minecraftdiamondsword .3 mm with all correct_v4 (Autodesk Fusion 360 design; units mm, degrees)
Autodesk Fusion 360 part; units mm, degrees
sketch "center" plane through (0, 0, 0) normal (0, 0, 1) x (1, 0, 0)
  line L0 (0, 22.6274) -> (2.8284, 19.799)
  line L1 (2.8284, 19.799) -> (5.6569, 22.6274)
  line L2 (5.6569, 22.6274) -> (2.8284, 25.4558)
  line L3 (2.8284, 25.4558) -> (0, 22.6274)
  line L4 (5.6569, 22.6274) -> (8.4853, 19.799)
  line L5 (8.4853, 19.799) -> (11.3137, 22.6274)
  line L6 (11.3137, 22.6274) -> (8.4853, 25.4558)
  line L7 (8.4853, 25.4558) -> (5.6569, 22.6274)
  line L8 (11.3137, 22.6274) -> (14.1421, 19.799)
  line L9 (14.1421, 19.799) -> (16.9706, 22.6274)
  line L10 (16.9706, 22.6274) -> (14.1421, 25.4558)
  line L11 (14.1421, 25.4558) -> (11.3137, 22.6274)
  line L12 (16.9706, 22.6274) -> (19.799, 19.799)
  line L13 (19.799, 19.799) -> (22.6274, 22.6274)
  line L14 (22.6274, 22.6274) -> (19.799, 25.4558)
  line L15 (19.799, 25.4558) -> (16.9706, 22.6274)
  line L16 (22.6274, 22.6274) -> (25.4558, 19.799)
  line L17 (25.4558, 19.799) -> (28.2843, 22.6274)
  line L18 (28.2843, 22.6274) -> (25.4558, 25.4558)
  line L19 (25.4558, 25.4558) -> (22.6274, 22.6274)
  line L20 (28.2843, 22.6274) -> (31.1127, 19.799)
  line L21 (31.1127, 19.799) -> (33.9411, 22.6274)
  line L22 (33.9411, 22.6274) -> (31.1127, 25.4558)
  line L23 (31.1127, 25.4558) -> (28.2843, 22.6274)
  line L24 (33.9411, 22.6274) -> (36.7696, 19.799)
  line L25 (36.7696, 19.799) -> (39.598, 22.6274)
  line L26 (39.598, 22.6274) -> (36.7696, 25.4558)
  line L27 (36.7696, 25.4558) -> (33.9411, 22.6274)
  line L28 (39.598, 22.6274) -> (42.4264, 19.799)
  line L29 (42.4264, 19.799) -> (45.2548, 22.6274)
  line L30 (45.2548, 22.6274) -> (42.4264, 25.4558)
  line L31 (42.4264, 25.4558) -> (39.598, 22.6274)
  line L32 (45.2548, 22.6274) -> (48.0833, 19.799)
  line L33 (48.0833, 19.799) -> (50.9117, 22.6274)
  line L34 (50.9117, 22.6274) -> (48.0833, 25.4558)
  line L35 (48.0833, 25.4558) -> (45.2548, 22.6274)
  line L36 (50.9117, 22.6274) -> (53.7401, 19.799)
  line L37 (53.7401, 19.799) -> (56.5685, 22.6274)
  line L38 (56.5685, 22.6274) -> (53.7401, 25.4558)
  line L39 (53.7401, 25.4558) -> (50.9117, 22.6274)
  line L40 (62.2254, 22.6274) -> (59.397, 25.4558)
  line L41 (70.7107, 25.4558) -> (67.8823, 22.6274)
  line L42 (90.5097, 22.6274) -> (87.6812, 25.4558)
  line L43 (62.2254, 22.6274) -> (65.0538, 19.799)
  line L44 (79.196, 22.6274) -> (76.3675, 25.4558)
  line L45 (84.8528, 22.6274) -> (87.6812, 19.799)
  line L46 (82.0244, 25.4558) -> (79.196, 22.6274)
  line L47 (76.3675, 25.4558) -> (73.5391, 22.6274)
  line L48 (87.6812, 25.4558) -> (84.8528, 22.6274)
  line L49 (73.5391, 22.6274) -> (76.3675, 19.799)
  line L50 (79.196, 22.6274) -> (82.0244, 19.799)
  line L51 (67.8823, 22.6274) -> (65.0538, 25.4558)
  line L52 (67.8823, 22.6274) -> (70.7107, 19.799)
  line L53 (76.3675, 19.799) -> (79.196, 22.6274)
  line L54 (59.397, 19.799) -> (62.2254, 22.6274)
  line L55 (56.5685, 22.6274) -> (59.397, 19.799)
  line L56 (59.397, 25.4558) -> (56.5685, 22.6274)
  line L57 (84.8528, 22.6274) -> (82.0244, 25.4558)
  line L58 (73.5391, 22.6274) -> (70.7107, 25.4558)
  line L59 (65.0538, 19.799) -> (67.8823, 22.6274)
  line L60 (87.6812, 19.799) -> (90.5097, 22.6274)
  line L61 (65.0538, 25.4558) -> (62.2254, 22.6274)
  line L62 (70.7107, 19.799) -> (73.5391, 22.6274)
  line L63 (82.0244, 19.799) -> (84.8528, 22.6274)
  dimension "d28" = 4
  dimension "d29" = 4
  dimension "d30" = 4
  dimension "d31" = 4
  dimension "d32" = 4
  dimension "d33" = 4
  dimension "d34" = 4
  dimension "d35" = 4
  dimension "d36" = 4
  dimension "d37" = 4
  dimension "d38" = 4
  dimension "d39" = 4
  dimension "d40" = 4
  dimension "d41" = 4
  dimension "d42" = 4
  dimension "d43" = 4
  dimension "d44" = 4
  dimension "d45" = 4
  dimension "d46" = 4
  dimension "d47" = 4
  dimension "d48" = 4
  dimension "d49" = 4
  dimension "d50" = 4
  dimension "d51" = 4
  dimension "d52" = 4
  dimension "d53" = 4
  dimension "d54" = 4
  dimension "d55" = 4
  dimension "d56" = 4
  dimension "d57" = 4
  dimension "d58" = 4
  dimension "d59" = 4
  measures "d28" distance of L0.start L0.end
  measures "d29" distance of L0.start L2.end
  measures "d30" distance of L1.end L4.end
  measures "d31" distance of L1.end L6.end
  measures "d32" distance of L5.end L8.end
  measures "d33" distance of L5.end L10.end
  measures "d34" distance of L9.end L12.end
  measures "d35" distance of L9.end L14.end
  measures "d36" distance of L13.end L16.end
  measures "d37" distance of L13.end L18.end
  measures "d38" distance of L20.end L21.end
  measures "d39" distance of L21.end L22.end
  measures "d40" distance of L21.end L24.end
  measures "d41" distance of L21.end L26.end
  measures "d42" distance of L25.end L28.end
  measures "d43" distance of L25.end L30.end
  measures "d44" distance of L29.end L32.end
  measures "d45" distance of L29.end L34.end
  measures "d46" distance of L33.end L36.end
  measures "d47" distance of L33.end L38.end
  measures "d48" distance of L54.start L37.end
  measures "d49" distance of L40.end L37.end
  measures "d50" distance of L43.end L40.start
  measures "d51" distance of L51.end L40.start
  measures "d52" distance of L52.end L41.end
  measures "d53" distance of L41.end L41.start
  measures "d54" distance of L47.end L49.end
  measures "d55" distance of L44.end L47.end
  measures "d56" distance of L44.start L50.end
  measures "d57" distance of L44.start L46.start
  measures "d58" distance of L45.end L42.start
  measures "d59" distance of L42.start L42.end
sketch "right" plane through (0, 0, 0) normal (0, 0, 1) x (1, 0, 0)
  line L0 (87.6812, 19.799) -> (84.8528, 22.6274)
  line L1 (25.4558, 19.799) -> (22.6274, 22.6274)
  line L2 (82.0244, 19.799) -> (84.8528, 16.9706)
  line L3 (33.9411, 16.9706) -> (36.7696, 19.799)
  line L4 (31.1127, 19.799) -> (33.9411, 16.9706)
  line L5 (33.9411, 22.6274) -> (31.1127, 19.799)
  line L6 (28.2843, 22.6274) -> (25.4558, 19.799)
  line L7 (16.9706, 22.6274) -> (14.1421, 19.799)
  line L8 (84.8528, 22.6274) -> (82.0244, 19.799)
  line L9 (67.8823, 16.9706) -> (70.7107, 19.799)
  line L10 (48.0833, 19.799) -> (45.2548, 22.6274)
  line L11 (65.0538, 19.799) -> (67.8823, 16.9706)
  line L12 (70.7107, 19.799) -> (67.8823, 22.6274)
  line L13 (53.7401, 19.799) -> (56.5685, 16.9706)
  line L14 (53.7401, 19.799) -> (50.9117, 22.6274)
  line L15 (50.9117, 22.6274) -> (48.0833, 19.799)
  line L16 (62.2254, 22.6274) -> (59.397, 19.799)
  line L17 (42.4264, 19.799) -> (39.598, 22.6274)
  line L18 (62.2254, 16.9706) -> (65.0538, 19.799)
  line L19 (31.1127, 19.799) -> (28.2843, 22.6274)
  line L20 (65.0538, 19.799) -> (62.2254, 22.6274)
  line L21 (76.3675, 19.799) -> (73.5391, 22.6274)
  line L22 (70.7107, 19.799) -> (73.5391, 16.9706)
  line L23 (67.8823, 22.6274) -> (65.0538, 19.799)
  line L24 (56.5685, 22.6274) -> (53.7401, 19.799)
  line L25 (59.397, 19.799) -> (62.2254, 16.9706)
  line L26 (45.2548, 16.9706) -> (48.0833, 19.799)
  line L27 (59.397, 19.799) -> (56.5685, 22.6274)
  line L28 (36.7696, 19.799) -> (39.598, 16.9706)
  line L29 (36.7696, 19.799) -> (33.9411, 22.6274)
  line L30 (42.4264, 19.799) -> (45.2548, 16.9706)
  line L31 (5.6569, 22.6274) -> (2.8284, 19.799)
  line L32 (16.9706, 16.9706) -> (19.799, 19.799)
  line L33 (19.799, 19.799) -> (16.9706, 22.6274)
  line L34 (79.196, 16.9706) -> (82.0244, 19.799)
  line L35 (73.5391, 16.9706) -> (76.3675, 19.799)
  line L36 (22.6274, 16.9706) -> (25.4558, 19.799)
  line L37 (25.4558, 19.799) -> (28.2843, 16.9706)
  line L38 (14.1421, 19.799) -> (11.3137, 22.6274)
  line L39 (28.2843, 16.9706) -> (31.1127, 19.799)
  line L40 (11.3137, 16.9706) -> (14.1421, 19.799)
  line L41 (84.8528, 16.9706) -> (87.6812, 19.799)
  line L42 (19.799, 19.799) -> (22.6274, 16.9706)
  line L43 (82.0244, 19.799) -> (79.196, 22.6274)
  line L44 (39.598, 22.6274) -> (36.7696, 19.799)
  line L45 (11.3137, 22.6274) -> (8.4853, 19.799)
  line L46 (45.2548, 22.6274) -> (42.4264, 19.799)
  line L47 (73.5391, 22.6274) -> (70.7107, 19.799)
  line L48 (56.5685, 16.9706) -> (59.397, 19.799)
  line L49 (48.0833, 19.799) -> (50.9117, 16.9706)
  line L50 (5.6569, 16.9706) -> (8.4853, 19.799)
  line L51 (22.6274, 22.6274) -> (19.799, 19.799)
  line L52 (2.8284, 19.799) -> (5.6569, 16.9706)
  line L53 (79.196, 22.6274) -> (76.3675, 19.799)
  line L54 (8.4853, 19.799) -> (11.3137, 16.9706)
  line L55 (8.4853, 19.799) -> (5.6569, 22.6274)
  line L56 (14.1421, 19.799) -> (16.9706, 16.9706)
  line L57 (76.3675, 19.799) -> (79.196, 16.9706)
  line L58 (8.4853, 19.799) -> (5.6569, 16.9706)
  line L59 (16.9706, 16.9706) -> (14.1421, 19.799)
  line L60 (45.2548, 16.9706) -> (48.0833, 14.1421)
  line L61 (28.2843, 16.9706) -> (25.4558, 19.799)
  line L62 (45.2548, 16.9706) -> (42.4264, 19.799)
  line L63 (33.9411, 16.9706) -> (31.1127, 19.799)
  line L64 (48.0833, 14.1421) -> (50.9117, 16.9706)
  line L65 (76.3675, 14.1421) -> (79.196, 16.9706)
  line L66 (65.0538, 19.799) -> (62.2254, 16.9706)
  line L67 (76.3675, 19.799) -> (73.5391, 16.9706)
  line L68 (62.2254, 16.9706) -> (65.0538, 14.1421)
  line L69 (59.397, 14.1421) -> (62.2254, 16.9706)
  line L70 (87.6812, 19.799) -> (84.8528, 16.9706)
  line L71 (70.7107, 14.1421) -> (73.5391, 16.9706)
  line L72 (53.7401, 19.799) -> (50.9117, 16.9706)
  line L73 (59.397, 19.799) -> (56.5685, 16.9706)
  line L74 (70.7107, 19.799) -> (67.8823, 16.9706)
  line L75 (73.5391, 16.9706) -> (70.7107, 19.799)
  line L76 (36.7696, 19.799) -> (33.9411, 16.9706)
  line L77 (82.0244, 19.799) -> (79.196, 16.9706)
  line L78 (82.0244, 14.1421) -> (84.8528, 16.9706)
  line L79 (22.6274, 16.9706) -> (19.799, 19.799)
  line L80 (56.5685, 16.9706) -> (53.7401, 19.799)
  line L81 (67.8823, 16.9706) -> (70.7107, 14.1421)
  line L82 (53.7401, 14.1421) -> (56.5685, 16.9706)
  line L83 (65.0538, 14.1421) -> (67.8823, 16.9706)
  line L84 (25.4558, 19.799) -> (22.6274, 16.9706)
  line L85 (39.598, 16.9706) -> (42.4264, 14.1421)
  line L86 (73.5391, 16.9706) -> (76.3675, 14.1421)
  line L87 (56.5685, 16.9706) -> (59.397, 14.1421)
  line L88 (50.9117, 16.9706) -> (48.0833, 19.799)
  line L89 (39.598, 16.9706) -> (36.7696, 19.799)
  line L90 (79.196, 16.9706) -> (82.0244, 14.1421)
  line L91 (84.8528, 16.9706) -> (82.0244, 19.799)
  line L92 (79.196, 16.9706) -> (76.3675, 19.799)
  line L93 (67.8823, 16.9706) -> (65.0538, 19.799)
  line L94 (42.4264, 14.1421) -> (45.2548, 16.9706)
  line L95 (50.9117, 16.9706) -> (53.7401, 14.1421)
  line L96 (62.2254, 16.9706) -> (59.397, 19.799)
  line L97 (31.1127, 19.799) -> (28.2843, 16.9706)
  line L98 (42.4264, 19.799) -> (39.598, 16.9706)
  line L99 (11.3137, 16.9706) -> (8.4853, 19.799)
  line L100 (19.799, 19.799) -> (16.9706, 16.9706)
  line L101 (14.1421, 19.799) -> (11.3137, 16.9706)
  dimension "d70" = 4
  dimension "d71" = 4
  dimension "d72" = 4
  dimension "d73" = 4
  dimension "d74" = 4
  dimension "d75" = 4
  dimension "d76" = 4
  dimension "d77" = 4
  dimension "d78" = 4
  dimension "d79" = 4
  dimension "d80" = 4
  dimension "d81" = 4
  dimension "d82" = 4
  dimension "d83" = 4
  dimension "d84" = 4
  dimension "d85" = 4
  dimension "d86" = 4
  dimension "d87" = 4
  dimension "d88" = 4
  dimension "d89" = 4
  dimension "d90" = 4
  dimension "d91" = 4
  dimension "d92" = 4
  dimension "d93" = 4
  dimension "d94" = 4
  dimension "d95" = 4
  dimension "d96" = 4
  dimension "d97" = 4
  dimension "d98" = 4
  dimension "d99" = 4
  dimension "d135" = 4
  dimension "d137" = 4
  dimension "d139" = 4
  dimension "d141" = 4
  dimension "d143" = 4
  dimension "d145" = 4
  dimension "d147" = 4
  dimension "d148" = 4
  dimension "d149" = 4
  dimension "d150" = 4
  dimension "d151" = 4
  dimension "d152" = 4
  dimension "d153" = 4
  dimension "d154" = 4
  dimension "d155" = 4
  dimension "d156" = 4
  dimension "d157" = 4
  dimension "d158" = 4
  dimension "d159" = 4
  dimension "d160" = 4
  dimension "d161" = 4
  measures "d70" distance of L50.start L31.end
  measures "d71" distance of L31.start L31.end
  measures "d72" distance of L40.start L45.end
  measures "d73" distance of L45.end L38.end
  measures "d74" distance of L7.end L32.start
  measures "d75" distance of L7.start L7.end
  measures "d76" distance of L32.end L36.start
  measures "d77" distance of L32.end L1.end
  measures "d78" distance of L37.end L4.start
  measures "d79" distance of L4.start L6.start
  measures "d80" distance of L4.start L3.start
  measures "d81" distance of L5.start L4.start
  measures "d82" distance of L28.end L3.end
  measures "d83" distance of L17.end L3.end
  measures "d84" distance of L26.start L17.start
  measures "d85" distance of L10.end L17.start
  measures "d86" distance of L49.end L10.start
  measures "d87" distance of L14.end L10.start
  measures "d88" distance of L13.end L13.start
  measures "d89" distance of L24.start L13.start
  measures "d90" distance of L18.start L16.end
  measures "d91" distance of L16.start L16.end
  measures "d92" distance of L11.start L9.start
  measures "d93" distance of L11.start L12.end
  measures "d94" distance of L9.end L22.end
  measures "d95" distance of L21.end L9.end
  measures "d96" distance of L34.start L21.start
  measures "d97" distance of L43.end L21.start
  measures "d98" distance of L0.start L2.end
  measures "d99" distance of L0.end L0.start
  measures "d135" distance of L45.end L50.start
  measures "d137" distance of L40.start L7.end
  measures "d139" distance of L32.end L32.start
  measures "d141" distance of L1.start L36.start
  measures "d143" distance of L4.start L3.start
  measures "d145" distance of L3.end L3.start
  measures "d147" distance of L28.end L17.start
  measures "d148" distance of L26.start L60.end
  measures "d149" distance of L10.start L26.start
  measures "d150" distance of L82.start L49.end
  measures "d151" distance of L13.start L49.end
  measures "d152" distance of L69.start L13.end
  measures "d153" distance of L13.end L16.end
  measures "d154" distance of L68.end L18.start
  measures "d155" distance of L18.start L11.start
  measures "d156" distance of L71.start L9.start
  measures "d157" distance of L9.end L9.start
  measures "d158" distance of L65.start L22.end
  measures "d159" distance of L21.start L22.end
  measures "d160" distance of L34.start L78.start
  measures "d161" distance of L34.start L2.start
sketch "left" plane through (0, 0, 0) normal (0, 0, 1) x (1, 0, 0)
  line L0 (11.3137, 28.2843) -> (8.4853, 25.4558)
  line L1 (48.0833, 25.4558) -> (50.9117, 22.6274)
  line L2 (14.1421, 25.4558) -> (11.3137, 28.2843)
  line L3 (76.3675, 25.4558) -> (73.5391, 28.2843)
  line L4 (14.1421, 25.4558) -> (16.9706, 22.6274)
  line L5 (11.3137, 22.6274) -> (14.1421, 25.4558)
  line L6 (53.7401, 25.4558) -> (50.9117, 28.2843)
  line L7 (33.9411, 22.6274) -> (36.7696, 25.4558)
  line L8 (33.9411, 28.2843) -> (31.1127, 25.4558)
  line L9 (53.7401, 25.4558) -> (56.5685, 22.6274)
  line L10 (70.7107, 25.4558) -> (73.5391, 22.6274)
  line L11 (50.9117, 22.6274) -> (53.7401, 25.4558)
  line L12 (87.6812, 25.4558) -> (84.8528, 28.2843)
  line L13 (82.0244, 25.4558) -> (79.196, 28.2843)
  line L14 (59.397, 25.4558) -> (56.5685, 28.2843)
  line L15 (8.4853, 25.4558) -> (11.3137, 22.6274)
  line L16 (56.5685, 28.2843) -> (53.7401, 25.4558)
  line L17 (25.4558, 25.4558) -> (22.6274, 28.2843)
  line L18 (5.6569, 28.2843) -> (2.8284, 25.4558)
  line L19 (22.6274, 22.6274) -> (25.4558, 25.4558)
  line L20 (8.4853, 25.4558) -> (5.6569, 28.2843)
  line L21 (28.2843, 28.2843) -> (25.4558, 25.4558)
  line L22 (45.2548, 22.6274) -> (48.0833, 25.4558)
  line L23 (16.9706, 28.2843) -> (14.1421, 25.4558)
  line L24 (16.9706, 22.6274) -> (19.799, 25.4558)
  line L25 (31.1127, 25.4558) -> (33.9411, 22.6274)
  line L26 (42.4264, 25.4558) -> (39.598, 28.2843)
  line L27 (19.799, 25.4558) -> (22.6274, 22.6274)
  line L28 (39.598, 28.2843) -> (36.7696, 25.4558)
  line L29 (36.7696, 25.4558) -> (39.598, 22.6274)
  line L30 (45.2548, 28.2843) -> (42.4264, 25.4558)
  line L31 (39.598, 22.6274) -> (42.4264, 25.4558)
  line L32 (36.7696, 25.4558) -> (33.9411, 28.2843)
  line L33 (31.1127, 25.4558) -> (28.2843, 28.2843)
  line L34 (42.4264, 25.4558) -> (45.2548, 22.6274)
  line L35 (70.7107, 25.4558) -> (67.8823, 28.2843)
  line L36 (73.5391, 28.2843) -> (70.7107, 25.4558)
  line L37 (59.397, 25.4558) -> (62.2254, 22.6274)
  line L38 (84.8528, 22.6274) -> (87.6812, 25.4558)
  line L39 (79.196, 22.6274) -> (82.0244, 25.4558)
  line L40 (79.196, 28.2843) -> (76.3675, 25.4558)
  line L41 (84.8528, 28.2843) -> (82.0244, 25.4558)
  line L42 (82.0244, 25.4558) -> (84.8528, 22.6274)
  line L43 (67.8823, 22.6274) -> (70.7107, 25.4558)
  line L44 (73.5391, 22.6274) -> (76.3675, 25.4558)
  line L45 (76.3675, 25.4558) -> (79.196, 22.6274)
  line L46 (62.2254, 28.2843) -> (59.397, 25.4558)
  line L47 (67.8823, 28.2843) -> (65.0538, 25.4558)
  line L48 (65.0538, 25.4558) -> (62.2254, 28.2843)
  line L49 (62.2254, 22.6274) -> (65.0538, 25.4558)
  line L50 (65.0538, 25.4558) -> (67.8823, 22.6274)
  line L51 (56.5685, 22.6274) -> (59.397, 25.4558)
  line L52 (19.799, 25.4558) -> (16.9706, 28.2843)
  line L53 (22.6274, 28.2843) -> (19.799, 25.4558)
  line L54 (2.8284, 25.4558) -> (5.6569, 22.6274)
  line L55 (5.6569, 22.6274) -> (8.4853, 25.4558)
  line L56 (50.9117, 28.2843) -> (48.0833, 25.4558)
  line L57 (28.2843, 22.6274) -> (31.1127, 25.4558)
  line L58 (48.0833, 25.4558) -> (45.2548, 28.2843)
  line L59 (25.4558, 25.4558) -> (28.2843, 22.6274)
  line L60 (42.4264, 25.4558) -> (39.598, 28.2843)
  line L61 (39.598, 28.2843) -> (42.4264, 31.1127)
  line L62 (42.4264, 31.1127) -> (45.2548, 28.2843)
  line L63 (45.2548, 28.2843) -> (42.4264, 25.4558)
  line L64 (48.0833, 25.4558) -> (45.2548, 28.2843)
  line L65 (45.2548, 28.2843) -> (48.0833, 31.1127)
  line L66 (48.0833, 31.1127) -> (50.9117, 28.2843)
  line L67 (50.9117, 28.2843) -> (48.0833, 25.4558)
  line L68 (53.7401, 25.4558) -> (50.9117, 28.2843)
  line L69 (50.9117, 28.2843) -> (53.7401, 31.1127)
  line L70 (53.7401, 31.1127) -> (56.5685, 28.2843)
  line L71 (56.5685, 28.2843) -> (53.7401, 25.4558)
  line L72 (59.397, 25.4558) -> (56.5685, 28.2843)
  line L73 (56.5685, 28.2843) -> (59.397, 31.1127)
  line L74 (59.397, 31.1127) -> (62.2254, 28.2843)
  line L75 (62.2254, 28.2843) -> (59.397, 25.4558)
  line L76 (65.0538, 25.4558) -> (62.2254, 28.2843)
  line L77 (62.2254, 28.2843) -> (65.0538, 31.1127)
  line L78 (65.0538, 31.1127) -> (67.8823, 28.2843)
  line L79 (67.8823, 28.2843) -> (65.0538, 25.4558)
  line L80 (70.7107, 25.4558) -> (67.8823, 28.2843)
  line L81 (67.8823, 28.2843) -> (70.7107, 31.1127)
  line L82 (70.7107, 31.1127) -> (73.5391, 28.2843)
  line L83 (73.5391, 28.2843) -> (70.7107, 25.4558)
  line L84 (76.3675, 25.4558) -> (73.5391, 28.2843)
  line L85 (73.5391, 28.2843) -> (76.3675, 31.1127)
  line L86 (76.3675, 31.1127) -> (79.196, 28.2843)
  line L87 (79.196, 28.2843) -> (76.3675, 25.4558)
  line L88 (82.0244, 25.4558) -> (79.196, 28.2843)
  line L89 (79.196, 28.2843) -> (82.0244, 31.1127)
  line L90 (82.0244, 31.1127) -> (84.8528, 28.2843)
  line L91 (84.8528, 28.2843) -> (82.0244, 25.4558)
  point P0 (0, 22.6274)
  dimension "d100" = 4
  dimension "d101" = 4
  dimension "d102" = 4
  dimension "d103" = 4
  dimension "d104" = 4
  dimension "d105" = 4
  dimension "d106" = 4
  dimension "d107" = 4
  dimension "d108" = 4
  dimension "d109" = 4
  dimension "d110" = 4
  dimension "d111" = 4
  dimension "d112" = 4
  dimension "d113" = 4
  dimension "d114" = 4
  dimension "d115" = 4
  dimension "d116" = 4
  dimension "d117" = 4
  dimension "d118" = 4
  dimension "d119" = 4
  dimension "d120" = 4
  dimension "d121" = 4
  dimension "d122" = 4
  dimension "d123" = 4
  dimension "d124" = 4
  dimension "d125" = 4
  dimension "d126" = 4
  dimension "d127" = 4
  dimension "d128" = 4
  dimension "d129" = 4
  dimension "d164" = 4
  dimension "d165" = 4
  dimension "d166" = 4
  dimension "d167" = 4
  dimension "d168" = 4
  dimension "d169" = 4
  dimension "d170" = 4
  dimension "d171" = 4
  dimension "d172" = 4
  dimension "d173" = 4
  dimension "d174" = 4
  dimension "d175" = 4
  dimension "d176" = 4
  dimension "d177" = 4
  dimension "d178" = 4
  dimension "d179" = 4
  measures "d100" distance of L54.end L18.end
  measures "d101" distance of L18.start L18.end
  measures "d102" distance of L5.start L0.end
  measures "d103" distance of L0.end L0.start
  measures "d104" distance of L4.end L2.start
  measures "d105" distance of L23.start L2.start
  measures "d106" distance of L19.start L24.end
  measures "d107" distance of L17.end L24.end
  measures "d108" distance of L8.end L57.start
  measures "d109" distance of L21.start L8.end
  measures "d110" distance of L8.end L7.start
  measures "d111" distance of L8.start L8.end
  measures "d112" distance of L29.end L7.end
  measures "d113" distance of L7.end L26.end
  measures "d114" distance of L26.start L22.start
  measures "d115" distance of L30.start L26.start
  measures "d116" distance of L1.end L1.start
  measures "d117" distance of L6.end L1.start
  measures "d118" distance of L9.end L6.start
  measures "d119" distance of L6.start L14.end
  measures "d120" distance of L37.end L14.start
  measures "d121" distance of L14.start L46.start
  measures "d122" distance of L43.start L47.end
  measures "d123" distance of L35.end L47.end
  measures "d124" distance of L10.end L10.start
  measures "d125" distance of L3.end L10.start
  measures "d126" distance of L3.start L39.start
  measures "d127" distance of L3.start L13.end
  measures "d128" distance of L12.start L38.start
  measures "d129" distance of L12.start L12.end
  measures "d164" distance of L26.start L26.end
  measures "d165" distance of L26.start L30.start
  measures "d166" distance of L1.start L30.start
  measures "d167" distance of L1.start L6.end
  measures "d168" distance of L6.start L6.end
  measures "d169" distance of L6.start L14.end
  measures "d170" distance of L14.start L14.end
  measures "d171" distance of L14.start L46.start
  measures "d172" distance of L47.end L46.start
  measures "d173" distance of L47.end L35.end
  measures "d174" distance of L10.start L35.end
  measures "d175" distance of L10.start L3.end
  measures "d176" distance of L3.start L3.end
  measures "d177" distance of L3.start L13.end
  measures "d178" distance of L13.start L13.end
  measures "d179" distance of L13.start L12.end
sketch "handle" plane through (0, 0, 0) normal (0, 0, 1) x (1, 0, 0)
  line L0 (8.4853, 31.1127) -> (11.3137, 28.2843)
  line L1 (11.3137, 28.2843) -> (8.4853, 25.4558)
  line L2 (8.4853, 25.4558) -> (5.6569, 28.2843)
  line L3 (5.6569, 28.2843) -> (8.4853, 31.1127)
  line L4 (8.4853, 19.799) -> (11.3137, 16.9706)
  line L5 (11.3137, 16.9706) -> (8.4853, 14.1421)
  line L6 (8.4853, 14.1421) -> (5.6569, 16.9706)
  line L7 (5.6569, 16.9706) -> (8.4853, 19.799)
  dimension "d130" = 4
  dimension "d131" = 4
  dimension "d132" = 4
  dimension "d133" = 4
  measures "d130" distance of L0.start L0.end
  measures "d131" distance of L0.start L2.end
  measures "d132" distance of L4.start L4.end
  measures "d133" distance of L4.start L6.end
sketch "guard" plane through (0, 0, 0) normal (0, 0, 1) x (1, 0, 0)
  line L0 (36.7696, 19.799) -> (39.598, 16.9706)
  line L1 (39.598, 16.9706) -> (36.7696, 14.1421)
  line L2 (36.7696, 14.1421) -> (33.9411, 16.9706)
  line L3 (33.9411, 16.9706) -> (36.7696, 19.799)
  line L4 (36.7696, 25.4558) -> (33.9411, 28.2843)
  line L5 (33.9411, 28.2843) -> (36.7696, 31.1127)
  line L6 (36.7696, 31.1127) -> (39.598, 28.2843)
  line L7 (39.598, 28.2843) -> (36.7696, 25.4558)
  line L8 (31.1127, 19.799) -> (33.9411, 16.9706)
  line L9 (33.9411, 16.9706) -> (31.1127, 14.1421)
  line L10 (31.1127, 14.1421) -> (28.2843, 16.9706)
  line L11 (28.2843, 16.9706) -> (31.1127, 19.799)
  line L12 (33.9411, 16.9706) -> (36.7696, 14.1421)
  line L13 (36.7696, 14.1421) -> (33.9411, 11.3137)
  line L14 (33.9411, 11.3137) -> (31.1127, 14.1421)
  line L15 (31.1127, 14.1421) -> (33.9411, 16.9706)
  line L16 (31.1127, 25.4558) -> (28.2843, 28.2843)
  line L17 (28.2843, 28.2843) -> (31.1127, 31.1127)
  line L18 (31.1127, 31.1127) -> (33.9411, 28.2843)
  line L19 (33.9411, 28.2843) -> (31.1127, 25.4558)
  line L20 (33.9411, 28.2843) -> (31.1127, 31.1127)
  line L21 (31.1127, 31.1127) -> (33.9411, 33.9411)
  line L22 (36.7696, 31.1127) -> (33.9411, 28.2843)
  line L23 (36.7696, 14.1421) -> (39.598, 11.3137)
  line L24 (39.598, 11.3137) -> (36.7696, 8.4853)
  line L25 (36.7696, 8.4853) -> (33.9411, 11.3137)
  line L26 (33.9411, 11.3137) -> (36.7696, 14.1421)
  line L27 (36.7696, 8.4853) -> (39.598, 5.6569)
  line L28 (39.598, 5.6569) -> (36.7696, 2.8284)
  line L29 (36.7696, 2.8284) -> (33.9411, 5.6569)
  line L30 (33.9411, 5.6569) -> (36.7696, 8.4853)
  line L31 (31.1127, 31.1127) -> (33.9411, 33.9411)
  line L32 (36.7696, 31.1127) -> (33.9411, 33.9411)
  line L33 (36.7696, 36.7696) -> (33.9411, 39.598)
  line L34 (33.9411, 39.598) -> (36.7696, 42.4264)
  line L35 (36.7696, 42.4264) -> (39.598, 39.598)
  line L36 (39.598, 39.598) -> (36.7696, 36.7696)
  line L37 (33.9411, 11.3137) -> (36.7696, 8.4853)
  line L38 (36.7696, 8.4853) -> (33.9411, 5.6569)
  line L39 (33.9411, 5.6569) -> (31.1127, 8.4853)
  line L40 (31.1127, 8.4853) -> (33.9411, 11.3137)
  line L41 (33.9411, 5.6569) -> (36.7696, 2.8284)
  line L42 (36.7696, 2.8284) -> (33.9411, 0)
  line L43 (33.9411, 0) -> (31.1127, 2.8284)
  line L44 (31.1127, 2.8284) -> (33.9411, 5.6569)
  line L45 (31.1127, 8.4853) -> (33.9411, 5.6569)
  line L46 (33.9411, 5.6569) -> (31.1127, 2.8284)
  line L47 (31.1127, 2.8284) -> (28.2843, 5.6569)
  line L48 (28.2843, 5.6569) -> (31.1127, 8.4853)
  line L49 (33.9411, 11.3137) -> (31.1127, 14.1421)
  line L50 (31.1127, 14.1421) -> (28.2843, 11.3137)
  line L51 (28.2843, 11.3137) -> (31.1127, 8.4853)
  line L52 (31.1127, 8.4853) -> (33.9411, 11.3137)
  line L53 (31.1127, 14.1421) -> (28.2843, 16.9706)
  line L54 (28.2843, 16.9706) -> (25.4558, 14.1421)
  line L55 (25.4558, 14.1421) -> (28.2843, 11.3137)
  line L56 (28.2843, 11.3137) -> (31.1127, 14.1421)
  line L57 (36.7696, 42.4264) -> (33.9411, 39.598)
  line L58 (31.1127, 36.7696) -> (33.9411, 39.598)
  line L59 (33.9411, 33.9411) -> (31.1127, 36.7696)
  line L60 (31.1127, 36.7696) -> (33.9411, 39.598)
  line L61 (33.9411, 33.9411) -> (31.1127, 31.1127)
  line L62 (31.1127, 31.1127) -> (28.2843, 33.9411)
  line L63 (28.2843, 33.9411) -> (31.1127, 36.7696)
  line L64 (31.1127, 31.1127) -> (28.2843, 33.9411)
  line L65 (28.2843, 33.9411) -> (25.4558, 31.1127)
  line L66 (25.4558, 31.1127) -> (28.2843, 28.2843)
  line L67 (28.2843, 28.2843) -> (31.1127, 31.1127)
  line L68 (33.9411, 39.598) -> (36.7696, 42.4264)
  line L69 (31.1127, 36.7696) -> (28.2843, 39.598)
  line L70 (28.2843, 39.598) -> (31.1127, 42.4264)
  line L71 (31.1127, 42.4264) -> (33.9411, 39.598)
  line L72 (33.9411, 39.598) -> (31.1127, 42.4264)
  line L73 (31.1127, 42.4264) -> (33.9411, 45.2548)
  line L74 (33.9411, 45.2548) -> (36.7696, 42.4264)
  line L75 (36.7696, 42.4264) -> (33.9411, 39.598)
  line L76 (36.7696, 31.1127) -> (39.598, 28.2843)
  line L77 (39.598, 28.2843) -> (36.7696, 25.4558)
  line L78 (36.7696, 25.4558) -> (33.9411, 28.2843)
  line L79 (33.9411, 33.9411) -> (36.7696, 36.7696)
  line L80 (33.9411, 39.598) -> (31.1127, 36.7696)
  line L81 (33.9411, 33.9411) -> (36.7696, 36.7696)
  line L82 (39.598, 33.9411) -> (36.7696, 31.1127)
  line L83 (33.9411, 33.9411) -> (36.7696, 36.7696)
  line L84 (39.598, 33.9411) -> (36.7696, 36.7696)
  line L85 (31.1127, 36.7696) -> (33.9411, 33.9411)
  line L86 (31.1127, 31.1127) -> (28.2843, 33.9411)
  line L87 (31.1127, 36.7696) -> (33.9411, 33.9411)
  line L88 (31.1127, 42.4264) -> (33.9411, 39.598)
  dimension "d180" = 4
  dimension "d181" = 4
  dimension "d182" = 4
  dimension "d183" = 4
  dimension "d184" = 4
  dimension "d185" = 4
  dimension "d186" = 4
  dimension "d187" = 4
  dimension "d188" = 4
  dimension "d189" = 4
  dimension "d190" = 4
  dimension "d191" = 4
  dimension "d192" = 4
  dimension "d193" = 4
  dimension "d194" = 4
  dimension "d195" = 4
  dimension "d197" = 4
  dimension "d200" = 4
  dimension "d202" = 4
  dimension "d203" = 4
  dimension "d204" = 4
  dimension "d205" = 4
  dimension "d206" = 4
  dimension "d207" = 4
  dimension "d208" = 4
  dimension "d209" = 4
  dimension "d210" = 4
  dimension "d211" = 4
  dimension "d212" = 4
  dimension "d213" = 4
  dimension "d215" = 4
  dimension "d217" = 4
  dimension "d219" = 4
  dimension "d220" = 4
  dimension "d221" = 4
  dimension "d222" = 4
  dimension "d223" = 4
  dimension "d234" = 4
  dimension "d235" = 4
  dimension "d236" = 4
  dimension "d237" = 4
  dimension "d246" = 4
  dimension "d247" = 4
  constraint coincident L33.end L34.start
  constraint coincident L34.end L35.start
  constraint coincident L17.end L18.start
  constraint perpendicular L33 L79
  constraint perpendicular L59 L80
  constraint perpendicular L33 L81
  constraint perpendicular L32 L82
  constraint perpendicular L36 L84
  constraint perpendicular L31 L85
  constraint perpendicular L65 L86
  constraint perpendicular L81 L87
  constraint perpendicular L57 L88
  measures "d180" distance of L0.start L0.end
  measures "d181" distance of L0.start L2.end
  measures "d182" distance of L4.start L4.end
  measures "d183" distance of L4.start L6.end
  measures "d184" distance of L8.start L2.end
  measures "d185" distance of L8.start L10.end
  measures "d186" distance of L2.end L1.end
  measures "d187" distance of L2.end L9.end
  measures "d188" distance of L16.start L16.end
  measures "d189" distance of L16.start L4.end
  measures "d190" distance of L4.end L17.end
  measures "d191" distance of L4.end L5.end
  measures "d192" distance of L1.end L23.end
  measures "d193" distance of L1.end L13.end
  measures "d194" distance of L24.end L27.end
  measures "d195" distance of L24.end L29.end
  measures "d197" distance of L21.end L17.end
  measures "d200" distance of L5.end L21.end
  measures "d202" distance of L33.start L33.end
  measures "d203" distance of L33.start L35.end
  measures "d204" distance of L13.end L24.end
  measures "d205" distance of L13.end L39.end
  measures "d206" distance of L29.end L28.end
  measures "d207" distance of L29.end L43.end
  measures "d208" distance of L39.end L29.end
  measures "d209" distance of L39.end L47.end
  measures "d210" distance of L13.end L9.end
  measures "d211" distance of L13.end L39.end
  measures "d212" distance of L9.end L10.end
  measures "d213" distance of L9.end L50.end
  measures "d215" distance of L33.end L34.end
  measures "d217" distance of L33.end L58.start
  measures "d219" distance of L33.end L58.start
  measures "d220" distance of L58.start L21.end
  measures "d221" distance of L58.start L62.end
  measures "d222" distance of L17.end L62.end
  measures "d223" distance of L17.end L16.end
  measures "d234" distance of L58.start L69.end
  measures "d235" distance of L58.start L33.end
  measures "d236" distance of L33.end L70.end
  measures "d237" distance of L33.end L34.end
  measures "d246" distance of L4.start L4.end
  measures "d247" distance of L4.start L6.end
extrude "Extrude10" add sketch "guard" sketch "right" sketch "center" sketch "left" sketch "handle" along normal blind 3 of sketch 2 of sketch 3 of sketch 4 of sketch 5
equation "d = 4 mm"
equation "d28 = d"
equation "d29 = d"
equation "d30 = d"
equation "d31 = d"
equation "d32 = d"
equation "d33 = d"
equation "d34 = d"
equation "d35 = d"
equation "d36 = d"
equation "d37 = d"
equation "d38 = d"
equation "d39 = d"
equation "d40 = d"
equation "d41 = d"
equation "d42 = d"
equation "d43 = d"
equation "d44 = d"
equation "d45 = d"
equation "d46 = d"
equation "d47 = d"
equation "d48 = d"
equation "d49 = d"
equation "d50 = d"
equation "d51 = d"
equation "d52 = d"
equation "d53 = d"
equation "d54 = d"
equation "d55 = d"
equation "d56 = d"
equation "d57 = d"
equation "d58 = d"
equation "d59 = d"
equation "d70 = d"
equation "d71 = d"
equation "d72 = d"
equation "d73 = d"
equation "d74 = d"
equation "d75 = d"
equation "d76 = d"
equation "d77 = d"
equation "d78 = d"
equation "d79 = d"
equation "d80 = d"
equation "d81 = d"
equation "d82 = d"
equation "d83 = d"
equation "d84 = d"
equation "d85 = d"
equation "d86 = d"
equation "d87 = d"
equation "d88 = d"
equation "d89 = d"
equation "d90 = d"
equation "d91 = d"
equation "d92 = d"
equation "d93 = d"
equation "d94 = d"
equation "d95 = d"
equation "d96 = d"
equation "d97 = d"
equation "d98 = d"
equation "d99 = d"
equation "d100 = d"
equation "d101 = d"
equation "d102 = d"
equation "d103 = d"
equation "d104 = d"
equation "d105 = d"
equation "d106 = d"
equation "d107 = d"
equation "d108 = d"
equation "d109 = d"
equation "d110 = d"
equation "d111 = d"
equation "d112 = d"
equation "d113 = d"
equation "d114 = d"
equation "d115 = d"
equation "d116 = d"
equation "d117 = d"
equation "d118 = d"
equation "d119 = d"
equation "d120 = d"
equation "d121 = d"
equation "d122 = d"
equation "d123 = d"
equation "d124 = d"
equation "d125 = d"
equation "d126 = d"
equation "d127 = d"
equation "d128 = d"
equation "d129 = d"
equation "d130 = d"
equation "d131 = d"
equation "d132 = d"
equation "d133 = d"
equation "d135 = d"
equation "d137 = d"
equation "d139 = d"
equation "d141 = d"
equation "d143 = d"
equation "d145 = d"
equation "d147 = d"
equation "d148 = d"
equation "d149 = d"
equation "d150 = d"
equation "d151 = d"
equation "d152 = d"
equation "d153 = d"
equation "d154 = d"
equation "d155 = d"
equation "d156 = d"
equation "d157 = d"
equation "d158 = d"
equation "d159 = d"
equation "d160 = d"
equation "d161 = d"
equation "d164 = d"
equation "d165 = d"
equation "d166 = d"
equation "d167 = d"
equation "d168 = d"
equation "d169 = d"
equation "d170 = d"
equation "d171 = d"
equation "d172 = d"
equation "d173 = d"
equation "d174 = d"
equation "d175 = d"
equation "d176 = d"
equation "d177 = d"
equation "d178 = d"
equation "d179 = d"
equation "d180 = d"
equation "d181 = d"
equation "d182 = d"
equation "d183 = d"
equation "d184 = d"
equation "d185 = d"
equation "d186 = d"
equation "d187 = d"
equation "d188 = d"
equation "d189 = d"
equation "d190 = d"
equation "d191 = d"
equation "d192 = d"
equation "d193 = d"
equation "d194 = d"
equation "d195 = d"
equation "d197 = d"
equation "d200 = d"
equation "d202 = d"
equation "d203 = d"
equation "d204 = d"
equation "d205 = d"
equation "d206 = d"
equation "d207 = d"
equation "d208 = d"
equation "d209 = d"
equation "d210 = d"
equation "d211 = d"
equation "d212 = d"
equation "d213 = d"
equation "d215 = d"
equation "d217 = d"
equation "d219 = d"
equation "d220 = d"
equation "d221 = d"
equation "d222 = d"
equation "d223 = d"
equation "d234 = d"
equation "d235 = d"
equation "d236 = d"
equation "d237 = d"
equation "StockHeight = 3 mm"
equation "d244 = StockHeight"
equation "d246 = d"
equation "d247 = d"
